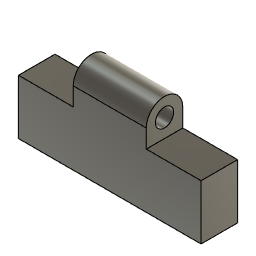
G13 - T PART (Autodesk Fusion 360 design; units mm, degrees)
Autodesk Fusion 360 part; units mm, degrees
sketch "Sketch1" plane through (0, 0, 0) normal (0, 0, 1) x (1, 0, 0)
  line L0 (0, 0) -> (-2.5418, 0)
  line L1 (-2.5418, 0) -> (-50, 0)
  line L2 (-50, 0) -> (-50, 100)
  line L3 (-50, 100) -> (0, 100)
  line L4 (0, 0) -> (0, 100)
  dimension "d1" = 50
  constraint coincident L0.start L4.start
  constraint horizontal L0
  constraint parallel L0 L1
  constraint perpendicular L1 L2
  constraint perpendicular L2 L3
  constraint perpendicular L3 L4
  measures "d1" distance of L2.end L3.end
extrude "Extrude1" add sketch "Sketch1" along normal blind 20 makes body 1
fillet "Fillet1" radius 10 2 edges at (0, 50, 0) (0, 50, 20) on bodies 1
sketch "Sketch2" plane through (0, 0, 0) normal (0, 0, 1) x (1, 0, 0)
  line L0 (-100, 0) -> (-130, 0)
  line L1 (-100, 0) -> (-100, 100)
  line L2 (-100, 100) -> (-130, 100)
  line L3 (-150, 70) -> (-130, 70)
  line L4 (-130, 30) -> (-150, 30)
  line L5 (-150, 30) -> (-150, 70)
  line L6 (-130, 70) -> (-130, 100)
  line L7 (-130, 30) -> (-130, 0)
  constraint horizontal L0
  constraint perpendicular L0 L1
  constraint perpendicular L1 L2
  constraint perpendicular L3 L5
  constraint perpendicular L2 L6
  constraint perpendicular L0 L7
extrude "Extrude2" add sketch "Sketch2" along normal blind 20 separate body makes body 2
fillet "Fillet2" radius 10 2 edges at (-150, 50, 20) (-150, 50, 0) on bodies 2
sketch "Sketch3" plane through (0, 70, 0) normal (0, 1, 0) x (-1, 0, 0)
  arc A0 (140, 0) -> (140, 20) centre (140, 10) ccw
  line L0 (140, 20) -> (130, 20)
  line L1 (130, 20) -> (130, 0)
  line L2 (130, 0) -> (140, 0)
  circle A1 centre (140, 10) radius 5
  dimension "d11" = 10
  constraint concentric A0 A1
  measures "d11" diameter of A1
extrude "Extrude3" cut sketch "Sketch3" against normal blind 40 contours A1 bodies 2
sketch "Sketch4" plane through (0, 0, 0) normal (1, 0, 0) x (0, 1, 0)
move_body "Move1" bodies 2 to x (0, 0, -1) y (0, 1, 0) z (1, 0, 0) at (0, 0, 0)
move_body "Move2" bodies 2 to x (0, -1, 0) y (1, 0, 0) z (0, 0, 1) at (0, 0, 0)
move_body "Move3" bodies 2 to x (1, 0, 0) y (0, 1, 0) z (0, 0, 1) at (0, 20, -100)
hidden bodies 1
